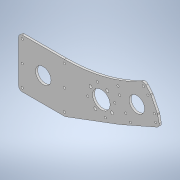
# Autodesk Inventor part: 関節3_側板右
Saved by Autodesk Inventor 2021 (Build 250183000, 183)
## iProperties
Created: 2022-02-03
Part Number: 関節3_側板右
Material: 一般
Document SubType Name: Modeling
Designer: hirohumi
Density: 1 g/cm^3
Appearance: 既定
Author: hirohumi
Autodesk Inventor part; units mm, degrees
ref_plane "YZ Plane" through (0, 0, 0) normal (1, 0, 0) x (0, 1, 0)
ref_plane "XZ Plane" through (0, 0, 0) normal (0, 1, 0) x (-1, 0, 0)
ref_plane "XY Plane" through (0, 0, 0) normal (0, 0, 1) x (1, 0, 0)
sketch "スケッチ1" plane through (0, 0, 0) normal (0, 0, 1) x (1, 0, 0)
  circle A0 centre (0, 0) radius 11.05
  line L0 (30, 30) -> (-30, 30) construction
  line L1 (-30, 30) -> (-30, -30) construction
  line L2 (-30, -30) -> (30, -30) construction
  line L3 (30, -30) -> (30, 30) construction
  line L4 (30, 30) -> (-30, -30) construction
  line L5 (-30, 30) -> (30, -30) construction
  circle A1 centre (-30, 30) radius 1.6
  circle A2 centre (30, 30) radius 1.6
  circle A3 centre (30, -30) radius 1.6
  circle A4 centre (-30, -30) radius 1.6
  circle A5 centre (-30, 0) radius 1.6
  circle A6 centre (30, 0) radius 1.6
  circle A7 centre (0, 300) radius 10 construction
  line L6 (0, 300) -> (82.4797, 11.5609) construction
  line L7 (0, 300) -> (132.9888, 31.0874)
  arc A8 (0, 0) -> (244.9763, 126.8336) centre (0, 300) ccw construction
  circle A9 centre (58.0974, 14.9896) radius 5 construction
  circle A10 centre (57.7518, 25.2915) radius 1.6
  line L8 (68.7491, -13.167) -> (107.2076, -2.1697) construction
  line L9 (63.5961, -4.2397) -> (106.8619, 8.1323) construction
  line L10 (58.0974, 14.9896) -> (106.8619, 8.1323) construction
  line L11 (101.3633, 27.3615) -> (63.5961, -4.2397) construction
  line L12 (101.3633, 27.3615) -> (58.0974, 14.9896) construction
  line L13 (96.2103, 36.2888) -> (68.7491, -13.167) construction
  line L14 (96.2103, 36.2888) -> (57.7518, 25.2915) construction
  circle A11 centre (82.4797, 11.5609) radius 12.55
  circle A12 centre (107.2076, -2.1697) radius 1.6
  circle A13 centre (107.2076, -2.1697) radius 4 construction
  line L15 (106.8619, 8.1323) -> (101.3633, 27.3615) construction
  circle A14 centre (101.3633, 27.3615) radius 1.25 construction
  circle A15 centre (63.5961, -4.2397) radius 1.25 construction
  line L16 (58.0974, 14.9896) -> (63.5961, -4.2397) construction
  line L17 (57.7518, 25.2915) -> (68.7491, -13.167) construction
  circle A16 centre (58.0974, 14.9896) radius 1.25 construction
  circle A17 centre (68.7491, -13.167) radius 1.6
  line L18 (57.7518, 25.2915) -> (107.2076, -2.1697) construction
  line L19 (107.2076, -2.1697) -> (96.2103, 36.2888) construction
  circle A18 centre (106.8619, 8.1323) radius 1.25 construction
  arc A19 (103.1758, 6.579) -> (103.327, 6.2604) centre (106.8619, 8.1323) ccw construction
  circle A20 centre (96.2103, 36.2888) radius 1.6
  line L20 (37.5, 43.7095) -> (22.5, 43.7095) construction
  line L21 (22.5, 43.7095) -> (22.5, -43.7095) construction
  line L22 (22.5, -43.7095) -> (37.5, -43.7095) construction
  line L23 (37.5, -43.7095) -> (37.5, 43.7095) construction
  line L24 (37.5, 43.7095) -> (22.5, -43.7095) construction
  line L25 (22.5, 43.7095) -> (37.5, -43.7095) construction
  circle A21 centre (132.9888, 31.0874) radius 23 construction
  arc A22 (-30, 35) -> (-35, 30) centre (-30, 30) ccw
  arc A23 (-35, -30) -> (-30, -35) centre (-30, -30) ccw
  arc A24 (30, -35) -> (31.7527, -34.6827) centre (30, -30) ccw
  arc A25 (110.3268, 27.1589) -> (111.2133, 23.683) centre (132.9888, 31.0874) ccw construction
  arc A26 (103.327, 6.2604) -> (103.1758, 6.579) centre (106.8619, 8.1323) ccw
  line L26 (108.7145, -5.8767) -> (31.7527, -34.6827)
  line L27 (30, -35) -> (-30, -35)
  line L28 (-35, -30) -> (-35, 30)
  line L29 (-30, 35) -> (30, 35)
  circle A27 centre (132.9888, 31.0874) radius 11.05
  line L30 (148.7243, 50.0253) -> (108.3874, 30.077) construction
  line L31 (108.3874, 30.077) -> (117.2533, 12.1495) construction
  line L32 (117.2533, 12.1495) -> (157.5902, 32.0978) construction
  line L33 (157.5902, 32.0978) -> (148.7243, 50.0253) construction
  line L34 (148.7243, 50.0253) -> (117.2533, 12.1495) construction
  line L35 (108.3874, 30.077) -> (157.5902, 32.0978) construction
  line L36 (142.0504, 57.8808) -> (106.1954, 40.149) construction
  line L37 (106.1954, 40.149) -> (123.9272, 4.294) construction
  line L38 (123.9272, 4.294) -> (159.7822, 22.0258) construction
  line L39 (159.7822, 22.0258) -> (142.0504, 57.8808) construction
  line L40 (142.0504, 57.8808) -> (123.9272, 4.294) construction
  line L41 (106.1954, 40.149) -> (159.7822, 22.0258) construction
  circle A28 centre (106.1954, 40.149) radius 1.6
  circle A29 centre (142.0504, 57.8808) radius 1.6
  circle A30 centre (148.7243, 50.0253) radius 1.6
  circle A31 centre (157.5902, 32.0978) radius 1.6
  circle A32 centre (159.7822, 22.0258) radius 1.6
  circle A33 centre (123.9272, 4.294) radius 1.6
  circle A34 centre (117.2533, 12.1495) radius 1.6
  circle A35 centre (108.3874, 30.077) radius 1.6
  arc A36 (145.8609, 61.1182) -> (139.7072, 62.2978) centre (142.0504, 57.8808) ccw
  arc A37 (153.2062, 52.2418) -> (152.5348, 53.2627) centre (148.7243, 50.0253) ccw
  arc A38 (161.7938, 17.4483) -> (164.6679, 23.0891) centre (159.7822, 22.0258) ccw
  arc A39 (30, 35) -> (139.7072, 62.2978) centre (30, 269.1002) ccw
  line L42 (145.8609, 61.1182) -> (152.5348, 53.2627)
  line L43 (153.2062, 52.2418) -> (162.0721, 34.3143)
  arc A40 (162.4759, 33.1611) -> (162.0721, 34.3143) centre (157.5902, 32.0978) ccw
  line L44 (162.4759, 33.1611) -> (164.6679, 23.0891)
  line L45 (161.7938, 17.4483) -> (108.7145, -5.8767)
  circle A41 centre (0, 0) radius 55 construction
  circle A42 centre (82.4797, 11.5609) radius 17.5 construction
  circle A43 centre (67.1801, 20.0563) radius 2.15
  circle A44 centre (90.9751, 26.8605) radius 2.15
  circle A45 centre (97.7793, 3.0655) radius 2.15
  circle A46 centre (73.9843, -3.7387) radius 2.15
  circle A47 centre (76.981, 30.7902) radius 1.6
  circle A48 centre (87.9783, -7.6683) radius 1.6
  circle A49 centre (101.709, 17.0596) radius 1.6
  circle A50 centre (63.2504, 6.0623) radius 1.6
  circle A51 centre (101.3633, 27.3615) radius 5 construction
  circle A52 centre (106.1954, 40.149) radius 5 construction
  circle A53 centre (123.9272, 4.294) radius 5 construction
  line L46 (101.7135, 37.9325) -> (119.4454, 2.0775) construction
  point P0 (82.4797, 11.5609)
  dimension "d71" = 10
  dimension "d72" = 10
  dimension "d0" = 22.1
  dimension "d1" = 60
  dimension "d2" = 60
  dimension "d3" = 3.2
  dimension "d4" = 3.2
  dimension "d5" = 3.2
  dimension "d6" = 3.2
  dimension "d7" = 3.2
  dimension "d8" = 3.2
  dimension "d9" = 20
  dimension "d10" = 300
  dimension "d12" = 25.1
  dimension "d13" = 20
  dimension "d14" = 45
  dimension "d15" = 40
  dimension "d16" = 40
  dimension "d17" = 3.2
  dimension "d18" = 2.5
  dimension "d19" = 2.5
  dimension "d20" = 3.2
  dimension "d21" = 3.2
  dimension "d22" = 2.5
  dimension "d23" = 2.5
  dimension "d24" = 3.2
  dimension "d26" = 8
  dimension "d27" = 8
  dimension "d28" = 10
  dimension "d29" = 15
  dimension "d30" = 46
  dimension "d31" = 23
  dimension "d33" = 5
  dimension "d34" = 5
  dimension "d35" = 5
  dimension "d36" = 5
  dimension "d37" = 22.1
  dimension "d38" = 45
  dimension "d39" = 20
  dimension "d40" = 40
  dimension "d41" = 40
  dimension "d42" = 3.2
  dimension "d43" = 3.2
  dimension "d44" = 3.2
  dimension "d45" = 3.2
  dimension "d46" = 3.2
  dimension "d47" = 3.2
  dimension "d48" = 3.2
  dimension "d49" = 3.2
  dimension "d50" = 5
  dimension "d52" = 5
  dimension "d54" = 5
  dimension "d56" = 5
  dimension "d59" = 110
  dimension "d60" = 35
  dimension "d61" = 4.3
  dimension "d62" = 4.3
  dimension "d63" = 4.3
  dimension "d64" = 4.3
  dimension "d65" = 3.2
  dimension "d66" = 3.2
  dimension "d67" = 3.2
  dimension "d68" = 3.2
  dimension "d70" = 10
  constraints: 94 end point, 52 centre point, 41 coincident, 31 point on circle, 24 midpoint, 18 tangent, 13 parallel, 10 perpendicular, 5 point on line, 2 horizontal, 1 vertical alignment, 8 other
  measures "d0" diameter of A0
  measures "d1" distance of L2.end L1.end
  measures "d2" distance of L1.end L0.end
  measures "d3" diameter of A1
  measures "d4" diameter of A2
  measures "d5" diameter of A3
  measures "d6" diameter of A4
  measures "d7" diameter of A5
  measures "d8" diameter of A6
  measures "d9" diameter of A7
  measures "d10" radius of A8
  measures "d12" diameter of A11
  measures "d13" distance of L10.start L9.start
  measures "d14" distance of L9.start L9.end
  measures "d15" distance of L8.start L8.end
  measures "d16" distance of L14.end L8.start
  measures "d17" diameter of A10
  measures "d18" diameter of A16
  measures "d19" diameter of A15
  measures "d20" diameter of A17
  measures "d21" diameter of A20
  measures "d22" diameter of A14
  measures "d23" diameter of A18
  measures "d24" diameter of A12
  measures "d26" diameter of A19
  measures "d27" diameter of A13
  measures "d28" diameter of A9
  measures "d29" distance of L22.end L21.end
  measures "d30" diameter of A21
  measures "d31" radius of A25
  measures "d33" radius of A22
  measures "d34" radius of A23
  measures "d35" radius of A24
  measures "d36" distance of L0.start L29.end
  measures "d37" diameter of A27
  measures "d38" distance of L32.end L31.end
  measures "d39" distance of L31.end L30.end
  measures "d40" distance of L38.end L37.end
  measures "d41" distance of L37.end L36.end
  measures "d42" diameter of A28
  measures "d43" diameter of A29
  measures "d44" diameter of A30
  measures "d45" diameter of A31
  measures "d46" diameter of A32
  measures "d47" diameter of A33
  measures "d48" diameter of A34
  measures "d49" diameter of A35
  measures "d50" radius of A37
  measures "d52" radius of A38
  measures "d54" radius of A36
  measures "d56" radius of A40
  measures "d59" diameter of A41
  measures "d60" diameter of A42
  measures "d61" diameter of A43
  measures "d62" diameter of A44
  measures "d63" diameter of A45
  measures "d64" diameter of A46
  measures "d65" diameter of A47
  measures "d66" diameter of A48
  measures "d67" diameter of A49
  measures "d68" diameter of A50
  measures "d70" diameter of A51
extrude "押し出し1" add sketch "スケッチ1" along normal blind 3 contours A39 A36 L42 A37 L43 A40 L44 A38 L45 L26 A24 L27 A23 L28 A22 L29 | A10 | A12 | A17 | A20
equation "\"d31\" = 0.5 * d30"
